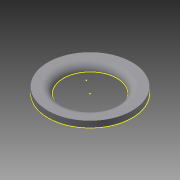
# Autodesk Inventor part: soporte2
Saved by Autodesk Inventor 2015 SP1 (Build 190203100, 203)
## iProperties
Created: 2015-06-29
Part Number: soporte2
Material: Genérico
Document SubType Name: Modeling
Designer: Javier
Density: 1 g/cm^3
Appearance: Valor por defecto
Author: Javier
Autodesk Inventor part; units mm, degrees
ref_plane "YZ Plane" through (0, 0, 0) normal (1, 0, 0) x (0, 1, 0)
ref_plane "XZ Plane" through (0, 0, 0) normal (0, 1, 0) x (-1, 0, 0)
ref_plane "XY Plane" through (0, 0, 0) normal (0, 0, 1) x (1, 0, 0)
sketch "Boceto1" plane through (0, 0, 0) normal (0, 0, 1) x (1, 0, 0)
  circle A0 centre (8.6443, 16.1632) radius 2.5 projected
  circle A1 centre (-13.8557, -6.3368) radius 2.5 projected
  circle A2 centre (8.6443, -28.8368) radius 2.5 projected
  circle A3 centre (31.1443, -6.3368) radius 2.5 projected
  circle A4 centre (8.6443, -6.3368) radius 17.5
  circle A5 centre (8.6443, -6.3368) radius 27.5
  point P0 (0, 0)
  dimension "d0" = 35
  dimension "d1" = 55
  constraints: 2 centre point, 1 coincident
  measures "d0" diameter of A4
  measures "d1" diameter of A5
extrude "Extrusión1" add sketch "Boceto1" along normal blind 4
sketch "Boceto2" plane through (8.6443, -6.3368, 4) normal (0, 0, 1) x (1, 0, 0)
  circle A0 centre (0, -22.5) radius 2.5 projected
  circle A1 centre (-22.5, 0) radius 2.5 projected
  circle A2 centre (0, 22.5) radius 2.5 projected
  circle A3 centre (22.5, 0) radius 2.5 projected
  point P0 (-8.6443, 6.3368)
extrude "Extrusión2" add sketch "Boceto2" against normal blind 2
fillet "Empalme1" radius 5 1 edges at (-8.8557, -6.3368, 4)
sketch "Boceto3" plane through (8.6443, -6.3368, 0) normal (0, 0, -1) x (-1, 0, 0)
  circle A0 centre (0, 0) radius 17.5 projected
  circle A1 centre (-22.5, 0) radius 2.5 projected
  circle A2 centre (0, -22.5) radius 2.5 projected
  circle A3 centre (22.5, 0) radius 2.5 projected
  circle A4 centre (0, 22.5) radius 2.5 projected
  circle A5 centre (0, 0) radius 27.5 projected
  point P0 (8.6443, 6.3368)
